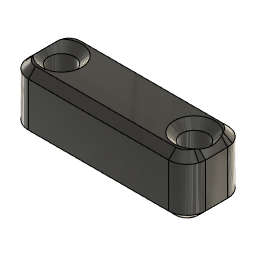
Belt_Fixture_Spacer (Autodesk Fusion 360 design; units mm, degrees)
Autodesk Fusion 360 part; units mm, degrees
note: some values were not read from the file. Set by a fixed rule: which sketch regions a step uses.
sketch "Sketch1" plane through (0, 0, 0) normal (0, 0, 1) x (1, 0, 0)
  circle A0 centre (0, 19) radius 1.75
  circle A1 centre (-18.04, 19) radius 1.75
  line L0 (0, 19) -> (3, 19) construction
  line L1 (-18.04, 19) -> (0, 19) construction
  line L2 (-9.02, 19) -> (-9.02, 15) construction
  line L3 (-21.04, 15) -> (3, 15)
  line L4 (3, 15) -> (3, 23)
  line L5 (3, 23) -> (-21.04, 23)
  line L6 (-21.04, 15) -> (-21.04, 23)
  point P0 (3, 23)
  point P1 (-21.04, 23)
  point P2 (-21.04, 15)
  dimension "d527" = 3
  dimension "d528" = 8
  constraint coincident A0.centre L0.start
  constraint coincident A1.centre L1.start
  constraint midpoint L1 L2.start
  constraint perpendicular L1 L2
  constraint symmetric L2 P0 P1
  constraint horizontal L3
  constraint vertical L4
  constraint horizontal L5
  constraint coincident P0 L4.end
  constraint coincident P2 L3.start
  constraint coincident L0.end L4
  constraint horizontal L0
  constraint midpoint L0.end L4
  constraint symmetric L2 L3.end P2
  constraint coincident P1 L5.end
  measures "d527" distance of A0.centre L0.end
  measures "d528" distance of L3.end P0
extrude "Extrude1" add sketch "Sketch1" against normal blind 8
fillet "Fillet1" radius 2.5 4 edges at (3, 15, -4) (-21.04, 15, -4) (-21.04, 23, -4) (3, 23, -4)
chamfer "Chamfer2" distance 1 angle 45 2 faces at (-6.4409, 15.9366, 0) (-6.4409, 15.9366, -8)
